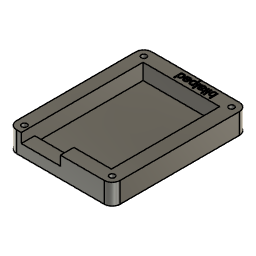
case (Autodesk Fusion 360 design; units mm, degrees)
Autodesk Fusion 360 part; units mm, degrees
sketch "Sketch1" plane through (0, 0, 0) normal (0, 0, 1) x (1, 0, 0)
  line L0 (0, 0) -> (48.5, 0)
  line L1 (48.5, 0) -> (48.5, 68.5)
  line L2 (48.5, 68.5) -> (0, 68.5)
  line L3 (0, 68.5) -> (0, 0)
  dimension "d1" = 48.5
  dimension "d2" = 68.5
  constraint horizontal L0
  constraint vertical L1
  constraint horizontal L2
  constraint vertical L3
  constraint coincident L0.start L3.end
  measures "d1" distance of L0.start L0.end
  measures "d2" distance of L0.start L2.end
sketch "Sketch2" plane through (0, 0, 0) normal (0, 0, 1) x (1, 0, 0)
  line L0 (-8, -8.5) -> (57.5, -8.5)
  line L1 (57.5, -8.5) -> (57.5, 77)
  line L2 (57.5, 77) -> (-8, 77)
  line L3 (-8, 77) -> (-8, -8.5)
  line L4 (48.5, 0) -> (48.5, 68.5)
  line L5 (48.5, 68.5) -> (0, 68.5)
  circle A0 centre (-3, -3.5) radius 1.7
  circle A1 centre (-3, 72) radius 1.7
  circle A2 centre (52.5, 72) radius 1.7
  circle A3 centre (52.5, -3.5) radius 1.7
  line L6 (0, 0) -> (48.5, 0)
  line L7 (48.5, 0) -> (48.5, 68.5)
  line L8 (48.5, 68.5) -> (0, 68.5)
  line L9 (0, 68.5) -> (0, 0)
  dimension "d3" = 65.5
  dimension "d4" = 85.5
  dimension "d5" = 68.5
  dimension "d6" = 48.5
  dimension "d7" = 3.4
  dimension "d8" = 5
  dimension "d9" = 5
  constraint horizontal L0
  constraint vertical L1
  constraint horizontal L2
  constraint vertical L3
  constraint horizontal L6
  constraint vertical L7
  constraint horizontal L8
  constraint vertical L9
  constraint coincident L4.end L5.start
  constraint coincident L6.start L9.end
  measures "d3" distance of L0.start L0.end
  measures "d4" distance of L0.start L2.end
  measures "d5" distance of L4.start L4.end
  measures "d6" distance of L4.end L5.end
  measures "d7" diameter of A0
  measures "d8" distance of L0 A0.centre
  measures "d9" distance of L3 A0.centre
extrude "Extrude1" add sketch "Sketch2" along normal blind 13
extrude "Extrude2" add sketch "Sketch1" along normal blind 3
sketch "Sketch3" plane through (0, 0, 13) normal (0, 0, 1) x (-1, 0, 0)
  circle A0 centre (-52.5, -72) radius 1.7
  circle A1 centre (3, 3.5) radius 1.7
  line L0 (0, 0) -> (0, -68.5)
  line L1 (0, -68.5) -> (-48.5, -68.5)
  line L2 (-48.5, -68.5) -> (-48.5, 0)
  line L3 (-48.5, 0) -> (0, 0)
  circle A2 centre (-52.5, 3.5) radius 1.7
  circle A3 centre (3, -72) radius 1.7
  line L4 (8, -77) -> (8, 8.5)
  line L5 (8, 8.5) -> (-57.5, 8.5)
  line L6 (-57.5, 8.5) -> (-57.5, -77)
  line L7 (-57.5, -77) -> (8, -77)
  line L8 (-24.75, 8.5) -> (0, 8.5)
  line L9 (0, 8.5) -> (0, 0)
  line L10 (0, 0) -> (-24.75, 0)
  line L11 (-24.75, 0) -> (-24.75, 8.5)
  constraint horizontal L8
  constraint vertical L9
  constraint horizontal L10
  constraint vertical L11
  constraint coincident L0.start L3.end
  constraint midpoint L5 L8.start
extrude "Extrude3" cut sketch "Sketch3" against normal blind 6 contours L3 L5 L8 L9 L10 L11
fillet "Fillet1" radius 5 4 edges at (57.5, 77, 6.5) (-8, 77, 6.5) (57.5, -8.5, 6.5) (-8, -8.5, 6.5)
sketch "Sketch4" plane through (0, 0, 13) normal (0, 0, 1) x (-1, 0, 0)
  circle A0 centre (3, -72) radius 1.7
  circle A1 centre (-52.5, 3.5) radius 1.7
  arc A2 (8, 3.5) -> (3, 8.5) centre (3, 3.5) ccw
  line L0 (3, 8.5) -> (0, 8.5)
  line L1 (0, 8.5) -> (0, -68.5)
  line L2 (0, -68.5) -> (-48.5, -68.5)
  line L3 (-48.5, -68.5) -> (-48.5, 0)
  line L4 (-48.5, 0) -> (-24.75, 0)
  line L5 (-24.75, 0) -> (-24.75, 8.5)
  line L6 (-24.75, 8.5) -> (-52.5, 8.5)
  arc A3 (-52.5, 8.5) -> (-57.5, 3.5) centre (-52.5, 3.5) ccw
  line L7 (-57.5, 3.5) -> (-57.5, -72)
  arc A4 (-57.5, -72) -> (-52.5, -77) centre (-52.5, -72) ccw
  line L8 (-52.5, -77) -> (3, -77)
  arc A5 (3, -77) -> (8, -72) centre (3, -72) ccw
  line L9 (8, -72) -> (8, 3.5)
  circle A6 centre (3, 3.5) radius 1.7
  circle A7 centre (-52.5, -72) radius 1.7
  line L10 (-41.0136, -73.9665) -> (-1.0136, -73.9665) construction
  line L11 (-1.0136, -73.9665) -> (-1.0136, -69.9665) construction
  line L12 (-1.0136, -69.9665) -> (-41.0136, -69.9665) construction
  line L13 (-41.0136, -69.9665) -> (-41.0136, -73.9665) construction
  dimension "d18" = 5
  text T0 "bilalpad" font "Arial" height 5 align left top in box 40 x 4 at (-41.0136, -73.9665) x (1, 0) y (0, 1) spacing 1
emboss "Emboss1" depth -2 profiles "Sketch4" section 1 text T0 onto face at (32.6667, 74.1667, 13)
